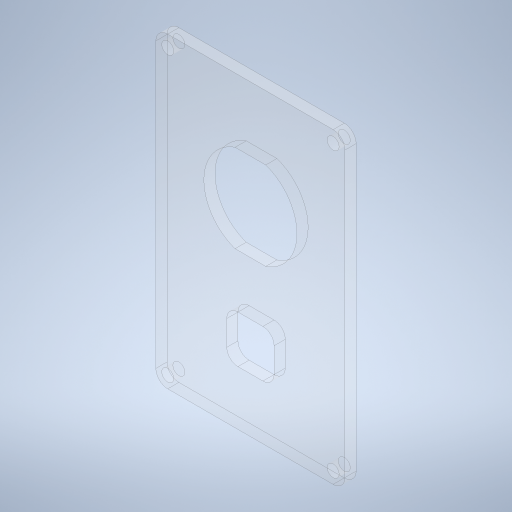
# Autodesk Inventor part: Cover
Saved by Autodesk Inventor 2023 (Build 270158000, 158)
## iProperties
Created: 2022-08-29
Part Number: Cover
Material: Generic
Document SubType Name: Modeling
Designer: swift
Density: 1 g/cm^3
Appearance: Clear - Light
Author: swift
Autodesk Inventor part; units mm, degrees
ref_plane "YZ Plane" through (0, 0, 0) normal (1, 0, 0) x (0, 1, 0)
ref_plane "XZ Plane" through (0, 0, 0) normal (0, 1, 0) x (-1, 0, 0)
ref_plane "XY Plane" through (0, 0, 0) normal (0, 0, 1) x (1, 0, 0)
sketch "Sketch1" plane through (0, 0, 0) normal (0, 0, 1) x (1, 0, 0)
  arc A0 (-3.175, 3.175) -> (0, 0) centre (0.0002, 3.1752) ccw projected
  line L0 (44.45, 0) -> (0, 0) projected
  arc A1 (44.45, 0) -> (47.625, 3.175) centre (44.4498, 3.1752) ccw projected
  line L1 (47.625, 79.375) -> (47.625, 3.175) projected
  arc A2 (47.625, 79.375) -> (44.45, 82.55) centre (44.4498, 79.3748) ccw projected
  line L2 (0, 82.55) -> (44.45, 82.55) projected
  arc A3 (0, 82.55) -> (-3.175, 79.375) centre (0.0002, 79.3748) ccw projected
  line L3 (-3.175, 3.175) -> (-3.175, 79.375) projected
  circle A4 centre (0, 3.175) radius 1.6 projected
  circle A5 centre (7.112, 4.191) radius 0.51 projected
  circle A6 centre (7.112, 9.271) radius 0.51 projected
  circle A7 centre (7.112, 6.731) radius 0.51 projected
  circle A8 centre (9.652, 6.731) radius 0.51 projected
  circle A9 centre (9.652, 4.191) radius 0.51 projected
  circle A10 centre (9.652, 9.271) radius 0.51 projected
  circle A11 centre (15.655, 10.499) radius 1.15 projected
  circle A12 centre (14.225, 36.449) radius 0.85 projected
  circle A13 centre (4.699, 60.198) radius 0.51 projected
  circle A14 centre (4.699, 57.658) radius 0.51 projected
  circle A15 centre (0, 79.375) radius 1.6 projected
  circle A16 centre (4.699, 62.738) radius 0.51 projected
  circle A17 centre (4.699, 65.278) radius 0.51 projected
  circle A18 centre (13.7, 69.341) radius 0.46 projected
  circle A19 centre (16.2, 69.341) radius 0.46 projected
  circle A20 centre (6.13, 72.051) radius 1.15 projected
  circle A21 centre (11.7, 69.341) radius 0.46 projected
  circle A22 centre (9.2, 69.341) radius 0.46 projected
  circle A23 centre (23.225, 13.209) radius 0.46 projected
  circle A24 centre (25.725, 13.209) radius 0.46 projected
  circle A25 centre (18.725, 13.209) radius 0.46 projected
  circle A26 centre (21.225, 13.209) radius 0.46 projected
  circle A27 centre (28.795, 10.499) radius 1.15 projected
  circle A28 centre (44.45, 3.175) radius 1.6 projected
  circle A29 centre (30.225, 36.449) radius 0.85 projected
  circle A30 centre (39.751, 57.531) radius 0.51 projected
  circle A31 centre (39.751, 60.071) radius 0.51 projected
  circle A32 centre (31.385, 69.341) radius 0.46 projected
  circle A33 centre (33.385, 69.341) radius 0.46 projected
  circle A34 centre (19.27, 72.051) radius 1.15 projected
  circle A35 centre (28.885, 69.341) radius 0.46 projected
  circle A36 centre (25.815, 72.051) radius 1.15 projected
  circle A37 centre (39.751, 65.151) radius 0.51 projected
  circle A38 centre (39.751, 62.611) radius 0.51 projected
  circle A39 centre (35.885, 69.341) radius 0.46 projected
  circle A40 centre (38.955, 72.051) radius 1.15 projected
  circle A41 centre (44.45, 79.375) radius 1.6 projected
  line L4 (19.2278, 19.1042) -> (19.2278, 22.8146) construction
  line L5 (20.234, 18.0978) -> (19.2662, 19.0663) construction
  line L6 (20.2568, 18.0747) -> (24.1988, 18.0747) construction
  line L7 (19.2662, 22.8525) -> (20.234, 23.821) construction
  line L8 (24.1988, 23.8441) -> (20.2568, 23.8441) construction
  line L9 (24.2216, 23.821) -> (25.1894, 22.8525) construction
  line L10 (25.2278, 22.8146) -> (25.2278, 19.1042) construction
  line L11 (25.1894, 19.0663) -> (24.2216, 18.0978) construction
  line L12 (19.2278, 23.8441) -> (25.2278, 23.8441) construction
  line L13 (25.2278, 23.8441) -> (25.2278, 18.0747) construction
  line L14 (25.2278, 18.0747) -> (19.2278, 18.0747) construction
  line L15 (19.2278, 18.0747) -> (19.2278, 23.8441) construction
  line L16 (19.2278, 20.9594) -> (25.2278, 20.9594) construction
  line L17 (22.2278, 23.8441) -> (22.2278, 18.0747) construction
  line L18 (15.8778, 27.3094) -> (28.5778, 27.3094)
  line L19 (28.5778, 27.3094) -> (28.5778, 14.6094)
  line L20 (28.5778, 14.6094) -> (15.8778, 14.6094)
  line L21 (15.8778, 14.6094) -> (15.8778, 27.3094)
  line L22 (15.8778, 27.3094) -> (28.5778, 14.6094) construction
  line L23 (28.5778, 27.3094) -> (15.8778, 14.6094) construction
  point P0 (22.2278, 20.9594)
  dimension "d0" = 12.7
  dimension "d1" = 12.7
  constraints: 24 end point, 7 midpoint, 4 parallel, 4 point on line, 2 horizontal, 2 perpendicular
  measures "d0" distance of L18.start L18.end
  measures "d1" distance of L18.end L19.end
extrude "Extrusion1" add sketch "Sketch1" along normal blind 3 contours L3 A3 L2 A2 L1 A1 L0 A0 | A5 | A6 | A7 | A8 | A9 | A10 | A11 | A12 | A13 | A14 | A16 | A17 | A18 | A19 | A20 | A21 | A22 | A23 | A24 | A25 | A26 | A27 | A29 | A30 | A31 | A32 | A33 | A34 | A35 | A36 | A37 | A38 | A39 | A40
fillet "Fillet1" radius 3 4 edges at (15.8778, 27.3094, 1.5) (28.5778, 27.3094, 1.5) (15.8778, 14.6094, 1.5) (28.5778, 14.6094, 1.5)
sketch "Sketch2" plane through (0, 0, 3) normal (0, 0, 1) x (1, 0, 0)
  line L0 (-3.175, 79.375) -> (-3.175, 3.175) construction
  arc A0 (-3.175, 3.175) -> (0, 0) centre (0.0002, 3.1752) ccw construction
  line L1 (0, 0) -> (44.45, 0) construction
  arc A1 (44.45, 0) -> (47.625, 3.175) centre (44.4498, 3.1752) ccw construction
  line L2 (47.625, 3.175) -> (47.625, 79.375) construction
  arc A2 (47.625, 79.375) -> (44.45, 82.55) centre (44.4498, 79.3748) ccw construction
  line L3 (44.45, 82.55) -> (0, 82.55) construction
  arc A3 (0, 82.55) -> (-3.175, 79.375) centre (0.0002, 79.3748) ccw construction
  line L4 (18.8778, 27.3094) -> (25.5778, 27.3094) construction
  arc A4 (28.5778, 24.3094) -> (25.5778, 27.3094) centre (25.5778, 24.3094) ccw construction
  line L5 (28.5778, 24.3094) -> (28.5778, 17.6094) construction
  arc A5 (25.5778, 14.6094) -> (28.5778, 17.6094) centre (25.5778, 17.6094) ccw construction
  line L6 (25.5778, 14.6094) -> (18.8778, 14.6094) construction
  arc A6 (15.8778, 17.6094) -> (18.8778, 14.6094) centre (18.8778, 17.6094) ccw construction
  line L7 (15.8778, 17.6094) -> (15.8778, 24.3094) construction
  arc A7 (18.8778, 27.3094) -> (15.8778, 24.3094) centre (18.8778, 24.3094) ccw construction
  circle A8 centre (44.45, 79.375) radius 1.6 construction
  circle A9 centre (44.45, 3.175) radius 1.6 construction
  circle A10 centre (0, 79.375) radius 1.6 construction
  circle A11 centre (0, 3.175) radius 1.6 construction
  circle A12 centre (22.225, 53.467) radius 12.4968
  line L8 (22.225, 82.55) -> (22.225, 0) construction
  line L9 (0, 0) -> (44.45, 0) construction
  line L10 (18.1055, 65.2653) -> (26.3445, 65.2653)
  line L11 (18.1055, 41.6687) -> (26.3445, 41.6687)
  line L12 (22.225, 65.9638) -> (22.225, 65.2653) construction
  line L13 (22.225, 41.6687) -> (22.225, 40.9702) construction
  dimension "d5" = 24.9936
  dimension "d6" = 53.467
  dimension "d7" = 23.5966
  dimension "d8" = 0.6985
  dimension "d9" = 0.6985
  constraints: 10 end point, 6 point on circle, 4 midpoint, 2 point on line, 1 centre point, 1 horizontal, 1 parallel, 1 vertical
  measures "d5" diameter of A12
  measures "d6" distance from line of L1 A12.centre
  measures "d7" distance between parallel lines of L11 L10
  measures "d8" distance of L12.start L12.end
  measures "d9" distance of L13.end L13.start
extrude "Extrusion2" cut sketch "Sketch2" against normal through all contours A12 L11 L10
equation "\"d1\" = d0"
equation "\"d9\" = d8"
body "Solid1"
